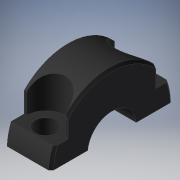
# Autodesk Inventor part: MBRAC45-2-10p2
Saved by Autodesk Inventor 2019 (Build 230136000, 136)
## iProperties
Created: 2024-03-05
Part Number: MBRAC45-2-10p2
Material: Generic
Catalog Web Link: www.cadenas.de
Description: MBRC, MBRAC-p2-Pulleys for Round Belts - Clamping
Vendor: MISUMI
Document SubType Name: Modeling
Designer: psAdmin
Manufacturer: MISUMI
Mass: 1.26287 g
Surface Area: 11.3165 cm^2
Volume: 1.26287 cm^3
Density: 1 g/cm^3
Appearance: PSOLRGB-175-175-175
Category: PARTsolutions
Company: MISUMI
Title: MBRAC45-2-10
Author: Cadenas PARTsolutions
Comments: Pulleys for Round Belts - Clamping
PSOL_IDENT_0: {$CADENAS_DATA/23d-libs/misumi/metric/52_belts_pulleys/mbrc_part2.prj},190 {VTYP=3D},{NB=MBRAC45-2-1
PSOL_IDENT_1: 0p2},{LINA=MBRAC45-2-10},{NN=MBRC, MBRAC-p2},{DATE=01.02.2024 02:39:30},{GEOMDATE=19.01.2024 07:24:4
PSOL_IDENT_2: 0},{VERSION=},{LINEID=30},{WBVAR=MAT,PD,DDS},{WBNUMERIC=PD,DDS}  {NB=MBRAC45-2-10p2},{LINA=MBRAC45-2
PSOL_IDENT_3: -10},{KT=DUMMY},{PN=MBRAC45-2-10},{TYPE=MBRAC},{MAT=2},{ST=Clear Anodizing},{AC=Hexagon Socket Head
PSOL_IDENT_4: Cap Screw (2Pcs.) Stainless Steel},{PD=45},{PD0=23,28,30,40,45,48,60,80},{R=2.0},{DDS=10.00},{DS0=5,
PSOL_IDENT_5: 6,6.35,8,10,11,12},{D=25},{D1=47},{D2=41},{L=20},{T=10},{LL=4.5},{X=9.0},{Y=4.5},{M=M4},{MM=4},{MMMI
PSOL_IDENT_6: N=3.242},{DD1=8.0},{DD2=4.5}
NB: MBRAC45-2-10p2
NN: MBRC, MBRAC-p2
NT: Pulleys for Round Belts - Clamping
NBSYN: $PN.p2
LINA: MBRAC45-2-10
CATALOG: Misumi
PN: MBRAC45-2-10
TYPE: MBRAC
MAT: 5052 Aluminum
ST: Clear Anodizing
AC: Hexagon Socket Head Cap Screw (2Pcs.) Stainless Steel
PD: 45
R: 2
DDS: 10
D: 25
D1: 47
D2: 41
L: 20
T: 10
LL: 4.5
X: 9
Y: 4.5
M: M4
DD1: 8
DD2: 4.5
SUPPLIER: MISUMI
ARTICLENO: MBRAC45-2-10p2
BOMINFO: MBRAC45-2-10
CREATOR: CADENAS GmbH
Autodesk Inventor part; units mm, degrees
sketch "Sketch_1" plane through (0, 0, 0) normal (0, 0, 1) x (1, 0, 0)
  line L0 (10, 0) -> (0, 0)
  line L1 (1, 5) -> (10, 5)
  line L2 (10, 5) -> (10, 12)
  line L3 (10, 12) -> (9.5, 12.5)
  line L4 (9.5, 12.5) -> (1, 12.5)
  line L5 (1, 12.5) -> (1, 5)
  constraints: 12 end point
revolve "Revolution1" add sketch "Sketch_1" angle 180 mid plane about axis through (10, 0, 0) along (-1, 0, 0)
sketch "Sketch_2" plane through (0, 0, 0) normal (0, 0, 1) x (1, 0, 0)
  line L0 (0, 0.5) -> (0, 0)
  line L1 (0, 0) -> (20, 0)
  line L2 (20, 0) -> (20, 0.5)
  line L3 (20, 0.5) -> (0, 0.5)
  constraints: 8 end point
extrude "Extrusion1" cut sketch "Sketch_2" along normal mid plane 50
sketch "Sketch_3" plane through (0, 0, 9) normal (0, 0, 1) x (1, 0, 0)
  line L0 (5.5, 12.5) -> (5.5, 0)
  line L1 (5.5, 0) -> (3.25, 0)
  line L2 (3.25, 0) -> (3.25, 4.5)
  line L3 (3.25, 4.5) -> (1.5, 4.5)
  line L4 (1.5, 4.5) -> (1.5, 12.5)
  line L5 (1.5, 12.5) -> (5.5, 12.5)
  line L6 (5.5, 12.5) -> (5.5, 0)
  constraints: 14 end point
revolve "Revolution2" cut sketch "Sketch_3" angle 360 about axis through (5.5, 12.5, 9) along (0, 1, 0)
sketch "Sketch_4" plane through (0, 0, -9) normal (0, 0, 1) x (1, 0, 0)
  line L0 (5.5, 12.5) -> (5.5, 0)
  line L1 (5.5, 0) -> (3.25, 0)
  line L2 (3.25, 0) -> (3.25, 4.5)
  line L3 (3.25, 4.5) -> (1.5, 4.5)
  line L4 (1.5, 4.5) -> (1.5, 12.5)
  line L5 (1.5, 12.5) -> (5.5, 12.5)
  line L6 (5.5, 12.5) -> (5.5, 0)
  constraints: 14 end point
revolve "Revolution3" cut sketch "Sketch_4" angle 360 about axis through (5.5, 12.5, -9) along (0, 1, 0)
sketch "Sketch_5" plane through (0, 0, 9) normal (0, 0, 1) x (1, 0, 0)
  line L0 (0, 17) -> (0, 4.5)
  line L1 (0, 4.5) -> (20, 4.5)
  line L2 (20, 4.5) -> (20, 17)
  line L3 (20, 17) -> (0, 17)
  constraints: 8 end point
extrude "Extrusion2" cut sketch "Sketch_5" along normal blind 25
sketch "Sketch_6" plane through (0, 0, -9) normal (0, 0, 1) x (1, 0, 0)
  line L0 (0, 17) -> (0, 4.5)
  line L1 (0, 4.5) -> (20, 4.5)
  line L2 (20, 4.5) -> (20, 17)
  line L3 (20, 17) -> (0, 17)
  constraints: 8 end point
extrude "Extrusion3" cut sketch "Sketch_6" against normal blind 25
ref_plane "part2_to_part1_XY" through (0, 0, 0) normal (1, 0, 0) x (0, 0, -1)
ref_plane "part2_to_part1_YZ" through (0, 0, 0) normal (0, 0, -1) x (0, 1, 0)
ref_plane "part2_to_part1_ZX" through (0, 0, 0) normal (0, 1, 0) x (1, 0, 0)
ref_plane "part2_to_screw1_XY" through (5.5, 4.5, 9) normal (0, 1, 0) x (1, 0, 0)
ref_plane "part2_to_screw1_YZ" through (5.5, 4.5, 9) normal (1, 0, 0) x (0, 0, -1)
ref_plane "part2_to_screw1_ZX" through (5.5, 4.5, 9) normal (0, 0, -1) x (0, 1, 0)
ref_plane "part2_to_screw2_XY" through (5.5, 4.5, -9) normal (0, 1, 0) x (1, 0, 0)
ref_plane "part2_to_screw2_YZ" through (5.5, 4.5, -9) normal (1, 0, 0) x (0, 0, -1)
ref_plane "part2_to_screw2_ZX" through (5.5, 4.5, -9) normal (0, 0, -1) x (0, 1, 0)
body "Solid1"
